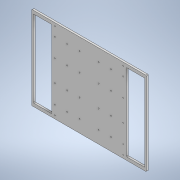
# Autodesk Inventor part: Chassis
Saved by Autodesk Inventor 2020.1 (Build 241239000, 239)
## iProperties
Created: 2019-11-14
Part Number: Chassis
Material: Generic
Document SubType Name: Modeling
Designer: Admin
Density: 1 g/cm^3
Appearance: Default
Author: Admin
Autodesk Inventor part; units mm, degrees
ref_plane "YZ Plane" through (0, 0, 0) normal (1, 0, 0) x (0, 1, 0)
ref_plane "XZ Plane" through (0, 0, 0) normal (0, 1, 0) x (-1, 0, 0)
ref_plane "XY Plane" through (0, 0, 0) normal (0, 0, 1) x (1, 0, 0)
sketch "Sketch1" plane through (0, 0, 0) normal (0, 0, 1) x (1, 0, 0)
  line L0 (-166.4634, 98.1707) -> (205.1366, 98.1707)
  line L1 (205.1366, 98.1707) -> (205.1366, -171.8293)
  line L2 (205.1366, -171.8293) -> (-166.4634, -171.8293)
  line L3 (-166.4634, -171.8293) -> (-166.4634, 98.1707)
  point P0 (0, 0)
  dimension "d0" = 371.6
  dimension "d1" = 270
  constraints: 8 end point, 2 parallel, 1 horizontal, 1 perpendicular
  measures "d0" distance of L0.start L0.end
  measures "d1" distance of L2.end L0.start
extrude "Extrusion1" add sketch "Sketch1" along normal blind 6
fillet "Fillet1" radius 2 1 edges at (-166.4634, 98.1707, 3)
fillet "Fillet2" radius 2 3 edges at (205.1366, 98.1707, 3) (205.1366, -171.8293, 3) (-166.4634, -171.8293, 3)
sketch "Sketch2" plane through (0, 0, 6) normal (0, 0, 1) x (1, 0, 0)
  line L0 (200.1366, -161.8293) -> (140.1366, -161.8293)
  line L1 (140.1366, -161.8293) -> (140.1366, 88.1707)
  line L2 (140.1366, 88.1707) -> (200.1366, 88.1707)
  line L3 (200.1366, 88.1707) -> (200.1366, -161.8293)
  line L4 (-101.4634, -161.8293) -> (-161.4634, -161.8293)
  line L5 (-161.4634, -161.8293) -> (-161.4634, 88.1707)
  line L6 (-161.4634, 88.1707) -> (-101.4634, 88.1707)
  line L7 (-101.4634, 88.1707) -> (-101.4634, -161.8293)
  line L8 (205.1366, -169.8293) -> (205.1366, 96.1707) projected
  line L9 (203.1366, 98.1707) -> (-164.4634, 98.1707) projected
  line L10 (-166.4634, 96.1707) -> (-166.4634, -169.8293) projected
  point P0 (0, 0)
  dimension "d6" = 60
  dimension "d7" = 60
  dimension "d8" = 250
  dimension "d9" = 250
  dimension "d10" = 65
  dimension "d11" = 10
  dimension "d12" = 10
  dimension "d13" = 65
  constraints: 16 end point, 4 parallel, 2 horizontal, 2 perpendicular
  measures "d6" distance of L0.start L0.end
  measures "d7" distance of L4.start L4.end
  measures "d8" distance of L2.end L0.start
  measures "d9" distance of L4.end L5.end
  measures "d10" distance between parallel lines of L8 L1
  measures "d11" distance between parallel lines of L9 L2
  measures "d12" distance between parallel lines of L9 L6
  measures "d13" distance between parallel lines of L10 L7
extrude "Extrusion2" cut sketch "Sketch2" against normal through all
fillet "Fillet3" radius 2 8 edges at (200.1366, -161.8293, 3) (-101.4634, -161.8293, 3) (-161.4634, -161.8293, 3) (140.1366, -161.8293, 3) (200.1366, 88.1707, 3) (-101.4634, 88.1707, 3) (-161.4634, 88.1707, 3) (140.1366, 88.1707, 3)
sketch "Sketch3" plane through (0, 0, 6) normal (0, 0, 1) x (1, 0, 0)
  circle A0 centre (-91.4634, 58.1707) radius 4.7928
  circle A1 centre (-51.4634, 58.1707) radius 10.8449
  circle A2 centre (-11.4634, 58.1707) radius 12.4429
  circle A3 centre (50.1366, 58.1707) radius 12.4797
  circle A4 centre (90.1366, 58.1707) radius 18.3008
  circle A5 centre (130.1366, 58.1707) radius 8.1337
  circle A6 centre (-91.4634, -1.8293) radius 12.8783
  circle A7 centre (-51.4634, -1.8293) radius 10.8449
  circle A8 centre (-11.4634, -1.8293) radius 12.4429
  circle A9 centre (50.1366, -1.8293) radius 10.8449
  circle A10 centre (90.1366, -1.8293) radius 10.1671
  circle A11 centre (130.1366, -1.8293) radius 18.5005
  line L0 (-101.4634, 86.1707) -> (-101.4634, -159.8293) projected
  line L1 (140.1366, -159.8293) -> (140.1366, 86.1707) projected
  line L2 (-159.4634, 88.1707) -> (-103.4634, 88.1707) projected
  line L3 (142.1366, 88.1707) -> (198.1366, 88.1707) projected
  circle A12 centre (-91.4634, -71.8293) radius 15.1871
  circle A13 centre (-91.4634, -131.8293) radius 15.3472
  circle A14 centre (-51.4634, -131.8293) radius 18.7949
  circle A15 centre (-51.4634, -71.8293) radius 21.2619
  circle A16 centre (-11.4634, -71.8293) radius 19.027
  circle A17 centre (-11.4634, -131.8293) radius 15.2356
  circle A18 centre (50.1366, -71.8293) radius 22.218
  circle A19 centre (50.1366, -131.8293) radius 15.9181
  circle A20 centre (90.1366, -71.8293) radius 11.5297
  circle A21 centre (130.1366, -71.8293) radius 12.0044
  circle A22 centre (90.1366, -131.8293) radius 9.1325
  circle A23 centre (130.1366, -131.8293) radius 9.1929
  line L4 (-164.4634, -171.8293) -> (203.1366, -171.8293) projected
  line L5 (-103.4634, -161.8293) -> (-159.4634, -161.8293) projected
  line L6 (198.1366, -161.8293) -> (142.1366, -161.8293) projected
  point P0 (0, 0)
  point P1 (140.1366, 86.1707)
  point P2 (-101.4634, -171.8293)
  point P3 (168.5366, -171.8293)
  dimension "d17" = 10
  dimension "d18" = 40
  dimension "d19" = 40
  dimension "d20" = 10
  dimension "d22" = 40
  dimension "d23" = 40
  dimension "d24" = 30
  dimension "d25" = 30
  dimension "d26" = 30
  dimension "d27" = 30
  dimension "d28" = 30
  dimension "d29" = 30
  dimension "d30" = 60
  dimension "d31" = 10
  dimension "d32" = 60
  dimension "d33" = 60
  dimension "d34" = 40
  dimension "d35" = 40
  dimension "d36" = 40
  dimension "d37" = 40
  dimension "d38" = 10
  dimension "d39" = 60
  dimension "d40" = 60
  dimension "d41" = 60
  dimension "d42" = 10
  dimension "d43" = 10
  dimension "d45" = 60
  dimension "d46" = 40
  dimension "d47" = 40
  dimension "d48" = 40
  dimension "d49" = 40
  dimension "d50" = 10
  dimension "d51" = 10
  dimension "d52" = 40
  dimension "d53" = 40
  dimension "d54" = 40
  dimension "d55" = 40
  dimension "d56" = 30
  dimension "d57" = 60
  dimension "d58" = 60
  dimension "d59" = 60
  dimension "d60" = 60
  dimension "d61" = 60
  dimension "d62" = 30
  dimension "d63" = 30
  dimension "d64" = 30
  dimension "d65" = 30
  dimension "d66" = 30
  constraints: 24 centre point, 1 other
  measures "d17" distance from line of L0 A0.centre
  measures "d18" distance of A0.centre A1.centre
  measures "d19" distance of A1.centre A2.centre
  measures "d22" distance of A5.centre A4.centre
  measures "d23" distance of A4.centre A3.centre
  measures "d24" distance from line of A0.centre L2
  measures "d25" distance from line of L2 A1.centre
  measures "d26" distance from line of L2 A2.centre
  measures "d27" distance from line of L3 A3.centre
  measures "d28" distance from line of L3 A4.centre
  measures "d29" distance from line of L3 A5.centre
  measures "d30" distance of A6.centre A0.centre
  measures "d31" distance from line of L0 A6.centre
  measures "d32" distance of A7.centre A1.centre
  measures "d33" distance of A2.centre A8.centre
  measures "d34" distance of A7.centre A6.centre
  measures "d35" distance of A8.centre A7.centre
  measures "d36" distance of A10.centre A11.centre
  measures "d37" distance of A9.centre A10.centre
  measures "d39" distance of A5.centre A11.centre
  measures "d40" distance of A4.centre A10.centre
  measures "d41" distance of A3.centre A9.centre
  measures "d42" distance from line of L0 A12.centre
  measures "d43" distance from line of L0 A13.centre
  measures "d45" distance of A13.centre A12.centre
  measures "d46" distance of A12.centre A15.centre
  measures "d47" distance of A16.centre A15.centre
  measures "d48" distance of A20.centre A18.centre
  measures "d49" distance of A21.centre A20.centre
  measures "d52" distance of A23.centre A22.centre
  measures "d53" distance of A22.centre A19.centre
  measures "d54" distance of A14.centre A17.centre
  measures "d55" distance of A13.centre A14.centre
  measures "d56" distance from line of L5 A13.centre
  measures "d57" distance of A15.centre A14.centre
  measures "d58" distance of A16.centre A17.centre
  measures "d59" distance of A19.centre A18.centre
  measures "d60" distance of A22.centre A20.centre
  measures "d61" distance of A23.centre A21.centre
  measures "d62" distance from line of L6 A19.centre
  measures "d63" distance from line of L6 A22.centre
  measures "d64" distance from line of L6 A23.centre
  measures "d65" distance from line of L5 A14.centre
  measures "d66" distance from line of L5 A17.centre
hole "Hole1" at (50.1366, -71.8293, 6) at (-91.4634, 58.1707, 6) at (-51.4634, 58.1707, 6) at (-11.4634, 58.1707, 6) at (-91.4634, -1.8293, 6) at (-51.4634, -1.8293, 6) at (-11.4634, -1.8293, 6) at (50.1366, -1.8293, 6) at (50.1366, 58.1707, 6) at (90.1366, 58.1707, 6) at (130.1366, 58.1707, 6) at (90.1366, -1.8293, 6) at (130.1366, -1.8293, 6) at (90.1366, -71.8293, 6) at (130.1366, -71.8293, 6) at (130.1366, -131.8293, 6) at (90.1366, -131.8293, 6) at (50.1366, -131.8293, 6) at (-91.4634, -71.8293, 6) at (-51.4634, -71.8293, 6) at (-11.4634, -71.8293, 6) at (-11.4634, -131.8293, 6) at (-51.4634, -131.8293, 6) at (-91.4634, -131.8293, 6) direction (0, 0, -1) diameter 3.3 end through all
sketch "Sketch4" plane through (0, 0, 6) normal (0, 0, 1) x (1, 0, 0)
  circle A0 centre (-91.4634, 88.1707) radius 1.5
  circle A1 centre (130.1366, 88.1707) radius 1.5
  circle A2 centre (130.1366, -161.8293) radius 1.5597
  circle A3 centre (-91.4634, -161.8293) radius 2.8966
  line L0 (203.1366, 98.1707) -> (-164.4634, 98.1707) projected
  line L1 (-101.4634, 86.1707) -> (-101.4634, -159.8293) projected
  line L2 (140.1366, -159.8293) -> (140.1366, 86.1707) projected
  line L3 (-164.4634, -171.8293) -> (203.1366, -171.8293) projected
  point P0 (0, 0)
  dimension "d74" = 3
  dimension "d75" = 10
  dimension "d76" = 10
  dimension "d77" = 10
  dimension "d78" = 3
  dimension "d79" = 10
  dimension "d80" = 10
  dimension "d81" = 10
  dimension "d82" = 10
  dimension "d83" = 10
  constraints: 4 centre point
  measures "d74" diameter of A0
  measures "d75" distance from line of L0 A0.centre
  measures "d76" distance from line of A0.centre L1
  measures "d77" distance from line of L2 A1.centre
  measures "d78" diameter of A1
  measures "d79" distance from line of L0 A1.centre
  measures "d80" distance from line of L1 A3.centre
  measures "d81" distance from line of L3 A3.centre
  measures "d82" distance from line of L3 A2.centre
  measures "d83" distance from line of L2 A2.centre
hole "Hole2" at (-91.4634, -161.8293, 6) at (130.1366, -161.8293, 6) at (-91.4634, 88.1707, 6) at (130.1366, 88.1707, 6) direction (0, 0, -1) diameter 3 end through all
body "Solid1"
